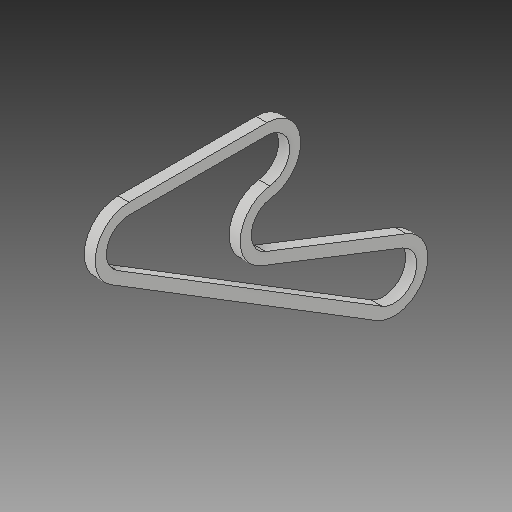
# Autodesk Inventor part: 15102898-16-P-0311
Saved by Autodesk Inventor 2017 (Build 210142000, 142)
## iProperties
Created: 2016-10-08
Part Number: 15102898-16-P-0311
Material: Generic
Document SubType Name: Modeling
Designer: gus
Density: 1 g/cm^3
Appearance: Default
Author: gus
Autodesk Inventor part; units mm, degrees
ref_plane "YZ Plane" through (0, 0, 0) normal (1, 0, 0) x (0, 1, 0)
ref_plane "XZ Plane" through (0, 0, 0) normal (0, 1, 0) x (-1, 0, 0)
ref_plane "XY Plane" through (0, 0, 0) normal (0, 0, 1) x (1, 0, 0)
sketch "Sketch1" plane through (0, 0, 0) normal (1, 0, 0) x (0, 1, 0)
  line L0 (0, 0) -> (0, -78.994)
  arc A0 (-32.2103, -80.9917) -> (0, -78.994) centre (-16.1671, -78.994) ccw
  arc A1 (-32.2103, -80.9917) -> (-63.3138, -77.1102) centre (-48.2535, -82.9893) ccw
  arc A2 (0, 0) -> (-29.9258, 8.4896) centre (-16.1671, 0) ccw
  line L1 (-63.3138, -77.1102) -> (-94.7528, -157.6461)
  line L2 (-29.9258, 8.4896) -> (-123.5718, -143.2774)
  arc A3 (-123.5718, -143.2774) -> (-94.7528, -157.6461) centre (-109.8131, -151.767) ccw
  line L3 (-32.2103, -80.9917) -> (-32.2103, -80.9917)
  dimension "d0" = 178.3334
  dimension "d1" = 78.994
  dimension "d3" = 92.3036
  dimension "d12" = 16.1671
  dimension "d14" = 88.9762
  constraints: 9 point on circle, 8 end point, 8 tangent, 4 centre point, 3 equal radius, 1 vertical
  measures "d0" distance of A2.centre A3.centre
  measures "d1" distance of A0.centre A2.centre
  measures "d3" distance of A3.centre A1.centre
  measures "d12" radius of A0
  measures "d14" distance of A2.centre A1.centre
sketch "Sketch2" plane through (0, 0, 0) normal (0, 0, 1) x (1, 0, 0)
  line L0 (-3.175, 3.175) -> (3.175, 3.175)
  line L1 (3.175, 3.175) -> (3.175, -3.175)
  line L2 (3.175, -3.175) -> (-3.175, -3.175)
  line L3 (-3.175, -3.175) -> (-3.175, 3.175)
  point P0 (0, 0)
  dimension "d5" = 6.35
  dimension "d6" = 6.35
  dimension "d7" = 3.175
  dimension "d8" = 3.175
  constraints: 8 end point, 2 parallel, 1 horizontal, 1 perpendicular
  measures "d5" distance of L0.start L0.end
  measures "d6" distance of L0.end L1.end
  measures "d7" distance from line of point (0, 0) L2
  measures "d8" distance from line of L1 point (0, 0)
sweep "Sweep2" add profiles "Sketch2" path "Sketch1" path curves L0 A0 A1 L1 A3 L2 A2
body "Solid2"
